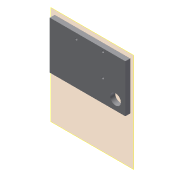
# Autodesk Inventor part: 10_MiniSPIM_Smarthponebase
Saved by Autodesk Inventor 2019 (Build 230136000, 136)
## iProperties
Created: 2019-10-13
Part Number: 10_MiniSPIM_Smarthponebase
Material: Generic
Document SubType Name: Modeling
Designer: diederichbenedict
Density: 1 g/cm^3
Appearance: Default
Author: diederichbenedict
Autodesk Inventor part; units mm, degrees
ref_plane "YZ Plane" through (0, 0, 0) normal (1, 0, 0) x (0, 1, 0)
ref_plane "XZ Plane" through (0, 0, 0) normal (0, 1, 0) x (-1, 0, 0)
ref_plane "XY Plane" through (0, 0, 0) normal (0, 0, 1) x (1, 0, 0)
ref_plane "Work Plane1" through (0, 0, 0) normal (0, 0, 1) x (1, 0, 0)
sketch "Sketch1" plane through (0, 0, 0) normal (0, 0, 1) x (1, 0, 0)
  circle A0 centre (35.6776, 53.4286) radius 1.65 construction
  circle A1 centre (91.3776, 7.2647) radius 7.5 construction
  circle A2 centre (73.1776, 24.5117) radius 1.65 construction
  circle A3 centre (73.1776, 56.6946) radius 1.65 construction
  circle A4 centre (75.9087, -63.7578) radius 1.65 construction
  circle A5 centre (1.8224, -63.7578) radius 1.65 construction
  line L0 (105.1776, 60.9647) -> (-1.8224, 60.9647) construction
  line L1 (-1.8224, 60.9647) -> (-1.8224, -66.5509) construction
  line L2 (-1.8224, -66.5509) -> (78.1776, -66.5509) construction
  line L3 (78.1776, -66.5509) -> (78.1776, -30.5509) construction
  line L4 (78.1776, -30.5509) -> (105.1776, -30.5509) construction
  line L5 (105.1776, -30.5509) -> (105.1776, 60.9647) construction
  line L6 (105.1776, 60.9647) -> (-1.8224, 60.9647)
  line L7 (-1.8224, 60.9647) -> (-1.8224, -6.5353)
  line L8 (-1.8224, -6.5353) -> (105.1776, -6.5353)
  line L9 (105.1776, -6.5353) -> (105.1776, 60.9647)
  circle A6 centre (91.3776, 7.2647) radius 7.5
  circle A7 centre (73.1776, 56.6946) radius 1.65 projected
  circle A8 centre (73.1776, 24.5117) radius 1.65 projected
  circle A9 centre (35.6776, 53.4286) radius 1.65 projected
  point P0 (0, 0)
  dimension "d0" = 13.8
  constraints: 8 end point, 2 parallel, 1 centre point, 1 coincident, 1 concentric, 1 horizontal, 1 perpendicular, 1 point on line
  measures "d0" distance from line of A1.centre L8
ref_plane "Work Plane2" through (-44.4224, -5.9353, 6.9) normal (0, 0, -1) x (0, 1, 0)
extrude "Extrusion1" add sketch "Sketch1" along normal up to surface (6.9 mm away)
body "Solid1"
